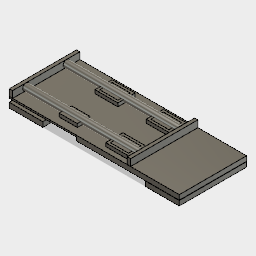
gantry v18 (Autodesk Fusion 360 design; units mm, degrees)
Autodesk Fusion 360 part; units mm, degrees
note: some values were not read from the file. Chosen so that the rebuilt part matches the saved one: which face or edge a step refers to.
box "BoxPrimitive1" add length 200 width 505 height 15 placed x (0, 0, -1) y (-1, 0, 0) z (0, 1, 0) at (505, 0, 0) makes body 1
sketch "Sketch2" plane through (0, 0, 0) normal (-1, 0, 0) x (0, 0, 1)
  line L0 (-200, 15) -> (-200, 0)
  line L1 (-200, 0) -> (0, 0)
  line L2 (0, 0) -> (0, 15)
  line L3 (0, 15) -> (-200, 15)
sketch "Sketch3" plane through (0, 15, 0) normal (0, 1, 0) x (-1, 0, 0)
  line L0 (-505, -200) -> (0, -200)
  line L1 (0, -200) -> (0, 0)
  line L2 (0, 0) -> (-505, 0)
  line L3 (-505, 0) -> (-505, -200)
  line L4 (-50, 0) -> (-50, -200)
  line L5 (0, -150) -> (-505, -150.2704)
  line L6 (-100, -200) -> (-100, 0)
  line L7 (-505, 0) -> (-455, 0)
  line L8 (-505, -200) -> (-455, -200)
  line L9 (-455, -200) -> (-455, 0)
  line L10 (-505, -200) -> (-405, -200)
  line L11 (-505, 0) -> (-405, 0)
  line L12 (-405, -200) -> (-405, 0)
  line L13 (0, -200) -> (-120, -200)
  line L14 (0, 0) -> (-120, 0)
  line L15 (0, -100) -> (-505, -100)
  line L16 (-119.9727, -185.65) -> (-187.9727, -185.6864)
  line L17 (-188, -134.6864) -> (-120, -134.65)
  line L18 (-187.9727, -185.6864) -> (-271.9727, -185.6864)
  line L19 (-187.9727, -134.6864) -> (-271.9727, -134.6864)
  line L20 (-119.9727, -185.65) -> (-120, -185.65)
  line L21 (-120, -134.65) -> (-119.9727, -134.65)
  line L22 (-119.9727, -134.65) -> (-119.9727, -185.65)
  line L23 (-130.0187, -185.65) -> (-120, -185.65)
  line L24 (-120, -134.65) -> (-130.0187, -134.65)
  line L25 (-120, -185.65) -> (-188, -185.65)
  line L26 (-188, -134.65) -> (-120, -134.65)
  line L27 (-120, -134.65) -> (-120, -185.65)
  line L28 (-120, -185.65) -> (-188, -185.65)
  line L29 (-188, -185.65) -> (-188, -134.65)
  line L30 (-188, -134.65) -> (-120, -134.65)
  line L31 (-120, -134.65) -> (-120, -185.65)
  line L32 (-120, -134.65) -> (-120, -65.35)
  line L33 (-120, -65.35) -> (-188, -65.35)
  line L34 (-120, -65.35) -> (-120, -14.35)
  line L35 (-120, -14.35) -> (-188, -14.35)
  line L36 (-188, -14.35) -> (-188, -65.35)
  line L37 (0, 0) -> (0, -50)
  line L38 (0, -50) -> (-505, -50.2637)
  dimension "d6" = 50
  dimension "d7" = 50
  dimension "d8" = 100
  dimension "d9" = 100
  dimension "d10" = 120
  dimension "d11" = 120
  dimension "d69" = 68
  dimension "d136" = 50
  measures "d6" distance of L2.end L7.end
  measures "d7" distance of L0.start L8.end
  measures "d8" distance of L0.start L10.end
  measures "d9" distance of L2.end L11.end
  measures "d10" distance of L0.end L13.end
  measures "d11" distance of L1.end L14.end
  measures "d69" distance of L34.end L35.end
  measures "d136" distance of L1.end L37.end
box "BoxPrimitive7" add length 51 width 68 height 10 placed x (0, 0, 1) y (1, 0, 0) z (0, 1, 0) at (120, 15, -185.65) separate body makes body 2
copy_body "CopyPasteBodies1" bodies 2 makes body 3
move_body "Move1" bodies 3 to x (1, 0, 0) y (0, 1, 0) z (0, 0, 1) at (0, 0, 120)
sketch "Sketch9" plane through (0, 0, 0) normal (0, 1, 0) x (1, 0, 0)
  line L0 (-50, 50) -> (-25, 50)
  line L1 (-25, 50) -> (-25, 25)
  line L2 (-25, 25) -> (-50, 25)
  line L3 (-50, 25) -> (-50, 50)
move_face "MoveFace1" by (0, 0, 0.3) 1 faces at (120, 18.3333, -31.65) on bodies 3
move_face "MoveFace2" by (0, 0, 0.03) 1 faces at (120, 18.3333, -31.65) on bodies 3
move_body "Move2" bodies 3 to x (1, 0, 0) y (0, 1, 0) z (0, 0, 1) at (0, 0, 0.3)
box "BoxPrimitive8" add length 51 width 68 height 10 placed x (0, 0, -1) y (-1, 0, 0) z (0, 1, 0) at (340, 15, -14.35) bodies 1
box "BoxPrimitive9" add length 51 width 68 height 10 placed x (0, 0, 1) y (1, 0, 0) z (0, 1, 0) at (272, 15, -185.65) bodies 1
sketch "Sketch15" plane through (0, 15, 0) normal (0, 1, 0) x (-1, 0, 0)
  line L0 (-272, -134.65) -> (-272, -185.65)
  line L1 (-272, -185.65) -> (-340, -185.65)
  line L2 (-340, -185.65) -> (-340, -134.65)
  line L3 (-340, -134.65) -> (-272, -134.65)
  line L4 (-340, -65.35) -> (-340, -14.35)
  line L5 (-340, -14.35) -> (-272, -14.35)
  line L6 (-272, -14.35) -> (-272, -65.35)
  line L7 (-272, -65.35) -> (-340, -65.35)
  line L8 (-505, -200) -> (0, -200)
  line L9 (0, -200) -> (0, 0)
  line L10 (0, 0) -> (-505, 0)
  line L11 (-505, 0) -> (-505, -200)
  line L12 (-306, -14.35) -> (-306, -65.35)
  line L13 (-306, -14.35) -> (-278, -14.35)
  line L14 (-306, -14.35) -> (-334, -14.35)
  line L15 (-340, -39.85) -> (-272, -39.85)
  line L16 (-340, -21.35) -> (-340, -14.35)
  line L17 (-340, -14.35) -> (-334, -14.35)
  line L18 (-272, -14.35) -> (-278, -14.35)
  line L19 (-272, -21.35) -> (-272, -14.35)
  line L20 (-306, -39.85) -> (-279, -39.85)
  line L21 (-279, -39.85) -> (-279, -21.35)
  line L22 (-279, -39.85) -> (-279, -58.35)
  line L23 (-279, -58.35) -> (-306, -58.35)
  line L24 (-306, -58.35) -> (-333, -58.35)
  line L25 (-333, -58.35) -> (-333, -39.85)
  line L26 (-333, -39.85) -> (-333, -21.35)
  line L27 (-333, -21.35) -> (-306, -21.35)
  line L28 (-279, -21.35) -> (-306, -21.35)
  line L29 (-279, -58.35) -> (-333, -58.35)
  line L30 (-333, -58.35) -> (-333, -21.35)
  line L31 (-333, -21.35) -> (-279, -21.35)
  line L32 (-279, -21.35) -> (-279, -58.35)
sketch "Sketch16" plane through (0, 0, 0) normal (0, 1, 0) x (1, 0, 0)
  line L0 (279, 58.35) -> (333, 58.35)
  line L1 (333, 58.35) -> (333, 21.35)
  line L2 (333, 21.35) -> (279, 21.35)
  line L3 (279, 21.35) -> (279, 58.35)
  point P0 (279, 58.35)
  point P1 (333, 21.35)
extrude "Extrude2" add sketch "Sketch16" along normal blind 10 separate body makes body 4
move_body "Move3" bodies 4 to x (1, 0, 0) y (0, 1, 0) z (0, 0, 1) at (0, 15, 0)
copy_body "CopyPasteBodies2" bodies 4 makes body 5
move_body "Move4" bodies 5 to x (1, 0, 0) y (0, 1, 0) z (0, 0, 1) at (0, 0, -120)
move_body "Align1" bodies 5 to x (1, 0, 0) y (0, 1, 0) z (0, 0, 1) at (-7, 0, -0.3)
move_body "Align2" bodies 5 to x (1, 0, 0) y (0, 1, 0) z (0, 0, 1) at (7, 0, 7)
move_body "Align3" bodies 5 to x (1, 0, 0) y (0, 1, 0) z (0, 0, 1) at (-7, 0, 0)
move_body "Move5" bodies 5 to x (1, 0, 0) y (0, 1, 0) z (0, 0, 1) at (0, 7, 0)
move_body "Move6" bodies 5 to x (1, 0, 0) y (0, 1, 0) z (0, 0, 1) at (0, 0, -7)
move_body "Move7" bodies 5 to x (1, 0, 0) y (0, 1, 0) z (0, 0, 1) at (7, 0, 0)
copy_body "CopyPasteBodies3" bodies 5 makes body 6
move_body "Move8" bodies 6 to x (1, 0, 0) y (0, 1, 0) z (0, 0, 1) at (-152.8, 0, 0)
move_body "Move9" bodies 6 to x (1, 0, 0) y (0, 1, 0) z (0, 0, 1) at (0, -7, 0)
move_body "Move10" bodies 5 to x (1, 0, 0) y (0, 1, 0) z (0, 0, 1) at (0, -7, 0)
copy_body "CopyPasteBodies4" bodies 6 makes body 7
move_body "Move11" bodies 7 to x (1, 0, 0) y (0, 1, 0) z (0, 0, 1) at (0, 0, 120.3)
move_body "Move12" bodies 7 to x (1, 0, 0) y (0, 1, 0) z (0, 0, 1) at (0.8, 0, 0)
move_body "Move13" bodies 6 to x (1, 0, 0) y (0, 1, 0) z (0, 0, 1) at (0.8, 0, 0)
sketch "Sketch18" plane through (0, 15, 0) normal (0, 1, 0) x (-1, 0, 0)
  line L0 (-272, -134.65) -> (-272, -185.65)
  line L1 (-272, -185.65) -> (-340, -185.65)
  line L2 (-340, -185.65) -> (-340, -134.65)
  line L3 (-340, -134.65) -> (-272, -134.65)
  line L4 (-340, -65.35) -> (-340, -14.35)
  line L5 (-340, -14.35) -> (-272, -14.35)
  line L6 (-272, -14.35) -> (-272, -65.35)
  line L7 (-272, -65.35) -> (-340, -65.35)
  line L8 (-505, -200) -> (0, -200)
  line L9 (0, -200) -> (0, 0)
  line L10 (0, 0) -> (-505, 0)
  line L11 (-505, 0) -> (-505, -200)
  line L12 (0, -200) -> (-300, -200)
  line L13 (-300, 0) -> (-290, 0)
  dimension "d153" = 10
  measures "d153" distance of L13.start L13.end
box "BoxPrimitive10" add length 200 width 10 height 20 placed x (0, 0, -1) y (-1, 0, 0) z (0, 1, 0) at (300, 15, 0) separate body makes body 8
move_body "Align4" bodies 8 to x (1, 0, 0) y (0, 1, 0) z (0, 0, 1) at (-290, 0, 0)
copy_body "CopyPasteBodies5" bodies 8 makes body 9
move_body "Move14" bodies 9 to x (1, 0, 0) y (0, 1, 0) z (0, 0, 1) at (350, 0, 0)
move_body "Move15" bodies 9 to x (1, 0, 0) y (0, 1, 0) z (0, 0, 1) at (0.3, 0, 0)
box "BoxPrimitive12" add length 200 width 100 height -15 placed x (0, 0, -1) y (-1, 0, 0) z (0, 1, 0) at (100, 15, 0) separate body makes body 10
move_body "Move16" bodies 10 to x (1, 0, 0) y (0, 1, 0) z (0, 0, 1) at (0, -15, 0)
box "BoxPrimitive13" add length 200 width 100 height 15 placed x (0, 0, 1) y (1, 0, 0) z (0, 1, 0) at (404.3014, 15, -200.3817) separate body makes body 11
move_body "Move17" bodies 11 to x (1, 0, 0) y (0, 1, 0) z (0, 0, 1) at (0, -30, 0)
cylinder "CylinderPrimitive1" add diameter 20 height 340.3 placed x (0, 0, 1) y (0, 1, 0) z (-1, 0, 0) at (350.3, 25, -160) separate body makes body 12
copy_body "CopyPasteBodies6" bodies 12 makes body 13
move_body "Move18" bodies 13 to x (1, 0, 0) y (0, 1, 0) z (0, 0, 1) at (0, 0, 120)
copy_body "CutPasteBodies1" bodies 1 removing the originals makes body 14 in component "Component"
copy_body "CutPasteBodies2" bodies 2 12 5 8 4 11 9 3 7 13 10 6 removing the originals makes body 15 makes body 16 makes body 17 makes body 18 makes body 19 makes body 20 makes body 21 makes body 22 makes body 23 makes body 24 makes body 25 makes body 26 in component "Component"
box "BoxPrimitive1'" cut length 40 width 200 height 10 placed x (0, 0, -1) y (-1, 0, 0) z (0, 1, 0) at (200, 0, 0) bodies 14 in component "Component"
box "BoxPrimitive1''" add length 40 width 200 height 10 placed x (0, 0, -1) y (-1, 0, 0) z (0, 1, 0) at (200, 0, 0) separate body makes body 27 in component "rail-su"
sketch "Sketch2 (2)" plane through (0, 10, 0) normal (0, 1, 0) x (-1, 0, 0) in component "rail-su"
  line L0 (-200, -40) -> (0, -40)
  line L1 (0, -40) -> (0, 0)
  line L2 (0, 0) -> (-200, 0)
  line L3 (-200, 0) -> (-200, -40)
  line L4 (0, -40) -> (-100, -40)
  line L5 (-100, 0) -> (-30.5, 0)
  line L6 (0, -40) -> (0, -19.5)
  line L7 (0, -19.5) -> (-200, -19.5)
  line L8 (-100, -40) -> (-100, 0)
  line L9 (-100, -19.5) -> (-30.5, -19.5)
  circle A0 centre (-30.5, -19.5) radius 9.975
  dimension "d195" = 69.5
  dimension "d196" = 20.5
  dimension "d197" = 200
  dimension "d198" = 69.5
  dimension "d199" = 19.95
  measures "d195" distance of L5.start L5.end
  measures "d196" distance of L0.end L6.end
  measures "d197" distance of L6.end L7.end
  measures "d198" distance of L9.start L9.end
  measures "d199" diameter of A0
extrude "Extrude1" cut sketch "Sketch2 (2)" against normal blind 10 contours L7 L9 A0 | L7 L9 A0 bodies 27 in component "rail-su"
sketch "Sketch3 (2)" plane through (0, 10, 0) normal (0, 1, 0) x (-1, 0, 0) in component "rail-su"
  circle A0 centre (-30.5, -19.5) radius 9.975
  line L0 (-200, -40) -> (0, -40)
  line L1 (0, -40) -> (0, 0)
  line L2 (0, 0) -> (-200, 0)
  line L3 (-200, 0) -> (-200, -40)
  line L4 (-100, -19.5) -> (-169.5, -19.5)
  point P0 (-100, -19.5)
  dimension "d202" = 69.5
  measures "d202" distance of P0 L4.end
cylinder "CylinderPrimitive1'" cut diameter 19.95 height -10 placed x (1, 0, 0) y (0, 0, -1) z (0, 1, 0) at (169.5, 10, -19.5) bodies 27 in component "rail-su"
cylinder "CylinderPrimitive2" cut diameter 18 height -10 placed x (1, 0, 0) y (0, 0, -1) z (0, 1, 0) at (100, 10, -20) bodies 27 in component "rail-su"
component "Component" placed x (1, 0, 0) y (0, 1, 0) z (0, 0, 1) at (0, 0, 0)
component "rail-su" placed x (1, 0, 0) y (0, 1, 0) z (0, 0, 1) at (0, 0, 0)
hidden bodies 22
